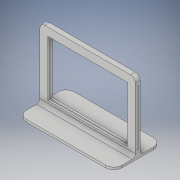
# Autodesk Inventor part: light_frame_v1
Saved by Autodesk Inventor 2019 (Build 230136000, 136)
## iProperties
Created: 2018-10-30
Part Number: light_frame_v1
Material: Generic
Document SubType Name: Modeling
Designer: Gianpietro
Density: 1 g/cm^3
Appearance: Default
Author: Gianpietro
Autodesk Inventor part; units mm, degrees
ref_plane "YZ Plane" through (0, 0, 0) normal (1, 0, 0) x (0, 1, 0)
ref_plane "XZ Plane" through (0, 0, 0) normal (0, 1, 0) x (-1, 0, 0)
ref_plane "XY Plane" through (0, 0, 0) normal (0, 0, 1) x (1, 0, 0)
sketch "Sketch1" plane through (0, 0, 0) normal (0, 0, 1) x (1, 0, 0)
  line L0 (-60, -45) -> (60, -45)
  line L1 (60, -45) -> (60, 45)
  line L2 (60, 45) -> (-60, 45)
  line L3 (-60, 45) -> (-60, -45)
  line L4 (-60, -45) -> (60, 45) construction
  line L5 (60, -45) -> (-60, 45) construction
  line L6 (-50, -35) -> (50, -35)
  line L7 (50, -35) -> (50, 35)
  line L8 (50, 35) -> (-50, 35)
  line L9 (-50, 35) -> (-50, -35)
  line L10 (-50, -35) -> (50, 35) construction
  line L11 (50, -35) -> (-50, 35) construction
  point P0 (0, 0)
  dimension "d0" = 120
  dimension "d1" = 90
  dimension "d2" = 100
  dimension "d3" = 70
  constraints: 24 end point, 4 midpoint, 4 parallel, 2 horizontal, 2 perpendicular
  measures "d0" distance of L2.end L1.end
  measures "d1" distance of L1.end L0.end
  measures "d2" distance of L8.end L7.end
  measures "d3" distance of L7.end L6.end
extrude "Extrusion1" add sketch "Sketch1" along normal blind 6
sketch "Sketch2" plane through (60, -45, 0) normal (1, 0, 0) x (0, 0, -1)
  line L0 (0, 0) -> (0, 90) projected
  line L1 (0, 90) -> (-6, 90) projected
  line L2 (-6, 0) -> (-6, 90) projected
  line L3 (0, 0) -> (-6, 0) projected
  line L4 (0, 45) -> (-3, 45)
  line L5 (-3.6, 9.9) -> (-2.4, 9.9)
  line L6 (-2.4, 9.9) -> (-2.4, 80.1)
  line L7 (-2.4, 80.1) -> (-3.6, 80.1)
  line L8 (-3.6, 80.1) -> (-3.6, 9.9)
  line L9 (-3.6, 9.9) -> (-2.4, 80.1) construction
  line L10 (-2.4, 9.9) -> (-3.6, 80.1) construction
  dimension "d6" = 3
  dimension "d7" = 1.2
  dimension "d8" = 70.2
  constraints: 14 end point, 2 horizontal, 2 midpoint, 2 parallel, 1 coincident, 1 perpendicular
  measures "d6" distance of L4.start L4.end
  measures "d7" distance of L7.end L6.end
  measures "d8" distance of L7.end L5.start
extrude "Extrusion2" cut sketch "Sketch2" against normal blind 120 contours L6 L5 L8 L7
sketch "Sketch3" plane through (-60, -45, 0) normal (0, -1, 0) x (1, 0, 0)
  line L0 (60, 0) -> (60, 3)
  line L1 (120, 33) -> (0, 33)
  line L2 (0, 33) -> (0, -27)
  line L3 (0, -27) -> (120, -27)
  line L4 (120, -27) -> (120, 33)
  line L5 (120, 33) -> (0, -27) construction
  line L6 (0, 33) -> (120, -27) construction
  dimension "d11" = 3
  dimension "d12" = 120
  dimension "d13" = 60
  constraints: 14 end point, 2 midpoint, 2 parallel, 1 coincident, 1 horizontal, 1 perpendicular, 1 vertical
  measures "d11" distance of L0.start L0.end
  measures "d12" distance of L3.end L2.end
  measures "d13" distance of L2.end L1.end
extrude "Extrusion3" add sketch "Sketch3" against normal blind 3
fillet "Fillet1" radius 4 2 edges at (0, -42, 6) (0, -42, 0)
fillet "Fillet2" radius 6 2 edges at (-60, 45, 3) (60, 45, 3)
fillet "Fillet3" radius 10 4 edges at (60, -43.5, 33) (60, -43.5, -27) (-60, -43.5, 33) (-60, -43.5, -27)
equation "\"d0\" = tot_w"
equation "\"d1\" = tot_h"
equation "\"d2\" = window_width"
equation "\"d3\" = window_height"
equation "\"d4\" = tot_t"
equation "\"d6\" = 0.5 * tot_t"
equation "\"d7\" = t + 2 * offset"
equation "\"d8\" = window_height + 2 * offset"
equation "\"d9\" = tot_w"
equation "\"d11\" = 0.5 * tot_t"
equation "\"d12\" = tot_w"
equation "\"d13\" = base_w"
equation "\"window_width\" = 100"
equation "\"window_height\" = 70"
equation "\"t\" = 1"
equation "\"offset\" = 0.1"
equation "\"tot_t\" = 6"
equation "\"tot_w\" = 120"
equation "\"tot_h\" = 90"
equation "\"base_w\" = 60"
body "Solid1"
